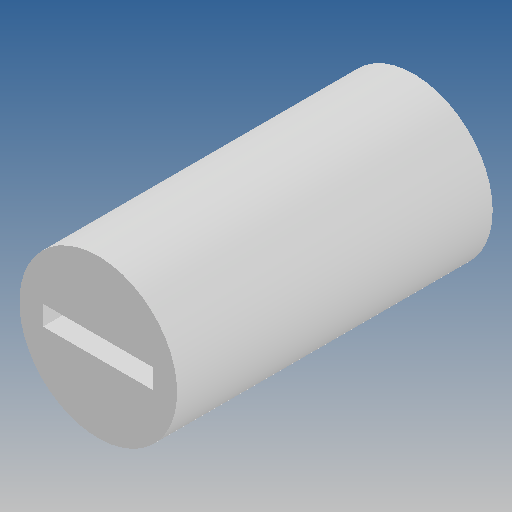
# Autodesk Inventor part: RollerMotorCoupler
Saved by Autodesk Inventor 2021 (Build 250183000, 183)
## iProperties
Created: 2022-09-08
Part Number: RollerMotorCoupler
Material: Generic
Document SubType Name: Modeling
Designer: Nathann
Density: 1 g/cm^3
Appearance: Default
Author: Nathann
Autodesk Inventor part; units mm, degrees
ref_plane "YZ Plane" through (0, 0, 0) normal (1, 0, 0) x (0, 1, 0)
ref_plane "XZ Plane" through (0, 0, 0) normal (0, 1, 0) x (-1, 0, 0)
ref_plane "XY Plane" through (0, 0, 0) normal (0, 0, 1) x (1, 0, 0)
sketch "Sketch1" plane through (0, 0, 0) normal (0, 0, 1) x (1, 0, 0)
  line L0 (1.5658, -2.5487) -> (1.5658, 2.559) projected
  arc A0 (1.5658, 2.559) -> (1.5824, -2.5487) centre (0, 0) ccw projected
  line L1 (1.5824, -2.5487) -> (1.5658, -2.5487) projected
  circle A1 centre (0, 0) radius 10
  circle A2 centre (0, 0) radius 3.1
  line L2 (1.7658, 2.5479) -> (1.7658, -2.5479)
  point P0 (0, 0)
  dimension "d0" = 20
  dimension "d1" = 6.2
  dimension "d2" = 0.2
  constraints: 2 centre point, 2 coincident, 2 end point, 2 point on circle, 1 vertical
  measures "d0" diameter of A1
  measures "d1" diameter of A2
  measures "d2" distance between parallel lines of L0 L2
extrude "Extrusion1" add sketch "Sketch1" against normal blind 10 contours A1 | A2 L2 picked at (2.2105, 0)
sketch "Sketch2" plane through (0, 0, 0) normal (0, 0, 1) x (1, 0, 0)
  circle A0 centre (0, 0) radius 3.1474
  circle A1 centre (0, 0) radius 10
  constraints: 2 centre point, 2 coincident
extrude "Extrusion2" add sketch "Sketch2" along normal blind 15
sketch "Sketch3" plane through (0, 0, 15) normal (0, 0, 1) x (1, 0, 0)
  line L0 (7, 1.25) -> (-7, 1.25)
  line L1 (-7, 1.25) -> (-7, -1.25)
  line L2 (-7, -1.25) -> (7, -1.25)
  line L3 (7, -1.25) -> (7, 1.25)
  circle A0 centre (0, 0) radius 10
  dimension "d7" = 2.5
  dimension "d8" = 14
  dimension "d9" = 1.25
  dimension "d10" = 7
  constraints: 8 end point, 2 parallel, 1 centre point, 1 coincident, 1 horizontal, 1 perpendicular
  measures "d7" distance of L2.end L0.start
  measures "d8" distance of L1.end L2.end
  measures "d9" distance from line of L0 point (0, 0)
  measures "d10" distance from line of L3 point (0, 0)
extrude "Extrusion3" add sketch "Sketch3" along normal blind 15
equation "\"d9\" = 0.5 * d7"
equation "\"d10\" = 0.5 * d8"
body "Solid1"
